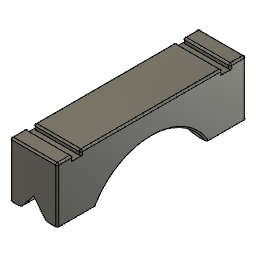
spine_bracket_for_torso_module (Autodesk Fusion 360 design; units mm, degrees)
Autodesk Fusion 360 part; units mm, degrees
box "BoxPrimitive1" add length 120 width 30 height 35 placed x (0, 0, -1) y (-1, 0, 0) z (0, 1, 0) at (30, 0, 0)
sketch "Sketch2" plane through (0, 0, 0) normal (0, 0, 1) x (1, 0, 0)
  line L0 (0, 35) -> (0, 0)
  line L1 (0, 0) -> (30, 0)
  line L2 (30, 0) -> (30, 35)
  line L3 (30, 35) -> (0, 35)
  line L4 (15, 0) -> (23, 0)
  line L5 (15, 0) -> (7, 0)
  line L6 (15, 0) -> (15, 10) construction
  line L7 (15, 10) -> (7, 0)
  line L8 (15, 10) -> (23, 0)
  dimension "d6" = 8
  dimension "d7" = 8
  dimension "d8" = 10
  constraint midpoint L1 L4.start
  constraint parallel L1 L4
  constraint parallel L1 L5
  constraint perpendicular L4 L6
  measures "d6" distance of L4.start L4.end
  measures "d7" distance of L4.start L5.end
  measures "d8" distance of L4.start L6.end
extrude "Extrude1" cut sketch "Sketch2" against normal blind 180.216 contours L1 L4 L5 L7 L8
sketch "Sketch3" plane through (30, 0, 0) normal (1, 0, 0) x (0, 0, -1)
  line L0 (0, 35) -> (0, 0)
  line L1 (0, 0) -> (120, 0)
  line L2 (120, 0) -> (120, 35)
  line L3 (120, 35) -> (0, 35)
  line L4 (0, 0) -> (25, 0)
  line L5 (120, 0) -> (95, 0)
  arc A0 (95, 0) -> (25, 0) centre (60, -20.625) ccw
  dimension "d11" = 25
  dimension "d12" = 25
  constraint coincident L0.end L1.start
  constraint perpendicular L0 L4
  constraint coincident L1.end L2.start
  constraint perpendicular L2 L5
  measures "d11" distance of L0.end L4.end
  measures "d12" distance of L1.end L5.end
extrude "Extrude2" cut sketch "Sketch3" against normal blind 49.649 contours L1 A0
sketch "Sketch4" plane through (0, 35, 0) normal (0, 1, 0) x (-1, 0, 0)
  line L0 (-30, -120) -> (0, -120)
  line L1 (0, -120) -> (0, 0)
  line L2 (0, 0) -> (-30, 0)
  line L3 (-30, 0) -> (-30, -120)
  line L4 (-30, 0) -> (-30, -10)
  line L5 (-30, -120) -> (-30, -110)
  line L6 (-30, -10) -> (0, -10)
  line L7 (0, -10) -> (0, -14)
  line L8 (0, -14) -> (-30, -14)
  line L9 (-30, -14) -> (-30, -10)
  line L10 (-30, -110) -> (0, -110)
  line L11 (0, -110) -> (0, -106)
  line L12 (0, -106) -> (-30, -106)
  line L13 (-30, -106) -> (-30, -110)
  dimension "d15" = 10
  dimension "d16" = 10
  dimension "d17" = 4
  dimension "d18" = 4
  constraint coincident L2.end L3.start
  constraint perpendicular L2 L4
  constraint coincident L0.start L3.end
  constraint perpendicular L0 L5
  constraint horizontal L6
  constraint vertical L7
  constraint horizontal L8
  constraint vertical L9
  constraint coincident L1 L7.end
  constraint horizontal L10
  constraint vertical L11
  constraint horizontal L12
  constraint vertical L13
  constraint coincident L1 L11.end
  measures "d15" distance of L2.end L4.end
  measures "d16" distance of L0.start L5.end
  measures "d17" distance of L4.end L8.end
  measures "d18" distance of L5.end L12.end
extrude "Extrude3" cut sketch "Sketch4" against normal blind 3 contours L1 L3 L6 L7 L8 L9
extrude "Extrude4" cut sketch "Sketch4" against normal blind 3 contours L1 L3 L10 L11 L12 L13
move_face "OffsetFaces1" offset -1 1 faces at (10, 33, -14)
move_face "OffsetFaces2" offset -1 1 faces at (10, 33, -106)
fillet "Fillet1" radius 1 1 edges at (30, 35, -60)
fillet "Fillet2" radius 1 3 edges at (30, 33, -105) (29.7071, 34.7071, -105) (14.5, 35, -105)
fillet "Fillet3" radius 1 1 edges at (30, 35, -115)
fillet "Fillet4" radius 1 3 edges at (30, 17, -120) (29.7071, 34.7071, -120) (14.5, 35, -120)
fillet "Fillet5" radius 1 3 edges at (0, 17, -120) (0, 34.7071, -119.7071) (0, 35, -114.5)
fillet "Fillet6" radius 1 5 edges at (0, 33, -110) (0.2929, 34.7071, -110) (15, 35, -110) (29.7071, 34.7071, -110) (30, 33, -110)
fillet "Fillet7" radius 1 3 edges at (0, 33, -105) (0, 34.7071, -104.7071) (0, 35, -59.5)
fillet "Fillet8" radius 1 5 edges at (0, 33, -15) (0.2929, 34.7071, -15) (15, 35, -15) (29.7071, 34.7071, -15) (30, 33, -15)
fillet "Fillet9" radius 1 1 edges at (30, 33.5, -10)
fillet "Fillet10" radius 1 1 edges at (0, 33.5, -10)
fillet "Fillet11" radius 1 5 edges at (30, 35, -4.5) (29.7071, 35, -9.7071) (15, 35, -10) (0.2929, 35, -9.7071) (0, 35, -4.5)
fillet "Fillet12" radius 1 5 edges at (0, 17, 0) (0.2929, 34.7071, 0) (15, 35, 0) (29.7071, 34.7071, 0) (30, 17, 0)
fillet "Fillet13" radius 1 1 edges at (30, 20, -60)
fillet "Fillet14" radius 1 1 edges at (0, 20, -60)
fillet "Fillet15" radius 3 1 edges at (23, 0, -12.5)
fillet "Fillet16" radius 3 1 edges at (7, 0, -12.5)
fillet "Fillet17" radius 3 1 edges at (23, 0, -107.5)
fillet "Fillet18" radius 3 1 edges at (7, 0, -107.5)
